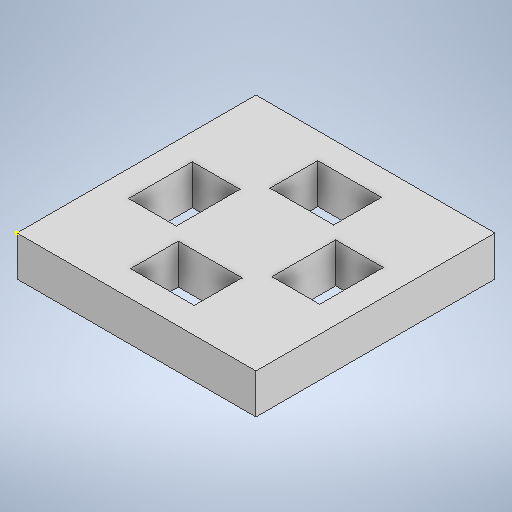
# Autodesk Inventor part: switch_test_v1
Saved by Autodesk Inventor 2025.4 (Build 294407000, 407)
## iProperties
Created: 2026-07-26
Part Number: switch_test_v1
Material: Generic
Document SubType Name: Modeling
Designer: Franchesca
Density: 1 g/cm^3
Appearance: Default
Author: Franchesca
Autodesk Inventor part; units mm, degrees
ref_plane "YZ Plane" through (0, 0, 0) normal (1, 0, 0) x (0, 1, 0)
ref_plane "XZ Plane" through (0, 0, 0) normal (0, 1, 0) x (-1, 0, 0)
ref_plane "XY Plane" through (0, 0, 0) normal (0, 0, 1) x (1, 0, 0)
sketch "Sketch1" plane through (0, 0, 0) normal (0, 1, 0) x (-1, 0, 0)
  point P0 (0, 0)
sketch "Sketch2" plane through (0, 0, 0) normal (0, 1, 0) x (-1, 0, 0)
  line L0 (0, 0) -> (-30, 0)
  line L1 (-30, 0) -> (-30, -30)
  line L2 (-30, -30) -> (0, -30)
  line L3 (0, -30) -> (0, 0)
  line L4 (0, -30) -> (-30, 0) construction
  line L5 (0, 0) -> (-30, -30) construction
  line L6 (-15, -15) -> (0, -15) construction
  line L7 (-15, -15) -> (-30, -15) construction
  line L8 (-15, -15) -> (-15, -30) construction
  line L9 (-15, -15) -> (-15, 0) construction
  line L10 (-15, -15) -> (-9.25, -15) construction
  line L11 (-15, -17.4158) -> (-15, -15) construction
  line L12 (-15, -15) -> (-15, -20.75) construction
  line L13 (-15, -15) -> (-15, -9.25) construction
  line L14 (-15, -15) -> (-9.25, -15) construction
  line L15 (-15, -15) -> (-20.75, -15) construction
  line L16 (-15, -20.75) -> (-9.25, -15) construction
  line L17 (-9.25, -15) -> (-9.25, -20.75) construction
  line L18 (-9.25, -20.75) -> (-15, -20.75) construction
  line L19 (-15, -20.75) -> (-20.75, -20.75) construction
  line L20 (-20.75, -20.75) -> (-20.75, -15) construction
  line L21 (-9.25, -15) -> (-9.25, -9.25) construction
  line L22 (-15, -9.25) -> (-9.25, -9.25) construction
  line L23 (-15, -9.25) -> (-20.75, -9.25) construction
  line L24 (-20.75, -9.25) -> (-20.75, -15) construction
  line L25 (-15, -9.25) -> (-11, -9.25) construction
  line L26 (-15, -9.25) -> (-19, -9.25) construction
  line L27 (-11, -9.25) -> (-19, -9.25)
  line L28 (-11, -9.25) -> (-11, -3.25)
  line L29 (-11, -3.25) -> (-19, -3.25)
  line L30 (-19, -3.25) -> (-19, -9.25)
  line L31 (-11, -20.75) -> (-19, -20.75)
  line L32 (-19, -20.75) -> (-19, -26.75)
  line L33 (-19, -26.75) -> (-11, -26.75)
  line L34 (-11, -26.75) -> (-11, -20.75)
  line L35 (-9.25, -9.25) -> (-9.25, -10.75)
  line L36 (-9.25, -20.75) -> (-9.25, -18.75)
  line L37 (-9.25, -18.75) -> (-9.25, -19.25)
  line L38 (-9.25, -18.75) -> (-9.25, -10.75)
  line L39 (-9.25, -10.75) -> (-3.25, -10.75)
  line L40 (-3.25, -10.75) -> (-3.25, -18.75)
  line L41 (-3.25, -18.75) -> (-9.25, -18.75)
  line L42 (-9.25, -19.25) -> (-20.75, -19.25) construction
  line L43 (-20.75, -19.25) -> (-20.75, -11.25)
  line L44 (-20.75, -11.25) -> (-26.75, -11.25)
  line L45 (-26.75, -11.25) -> (-26.75, -19.25)
  line L46 (-26.75, -19.25) -> (-20.75, -19.25)
  line L47 (-9.25, -18.75) -> (-11.75, -18.75) construction
  line L48 (-11.75, -18.75) -> (-11.75, -10.75) construction
  line L49 (-11.75, -10.75) -> (-9.25, -10.75) construction
  line L50 (-20.75, -19.25) -> (-18.25, -19.25) construction
  line L51 (-18.25, -19.25) -> (-18.25, -11.25) construction
  line L52 (-18.25, -11.25) -> (-20.75, -11.25) construction
  line L53 (-9.25, -10.75) -> (-9.25, -11.75) construction
  line L54 (-9.25, -11.75) -> (-11.75, -11.75) construction
  line L55 (-20.75, -11.25) -> (-20.75, -11.75) construction
  line L56 (-20.75, -11.75) -> (-18.25, -11.75) construction
  line L57 (-11.75, -18.75) -> (-20.75, -18.75) construction
  line L58 (-18.25, -18.75) -> (-18.25, -11.75) construction
  line L59 (-15, -18.75) -> (-14.25, -18.75) construction
  line L60 (-15, -18.75) -> (-15.75, -18.75) construction
  line L61 (-11.75, -18.75) -> (-11.75, -11.75)
  line L62 (-11.75, -18.75) -> (-14.25, -18.75)
  line L63 (-11.75, -11.75) -> (-14.25, -11.75)
  line L64 (-14.25, -18.75) -> (-14.25, -11.75)
  line L65 (-15.75, -18.75) -> (-18.25, -18.75)
  line L66 (-18.25, -18.75) -> (-18.25, -11.75)
  line L67 (-18.25, -11.75) -> (-15.75, -11.75)
  line L68 (-15.75, -11.75) -> (-15.75, -18.75)
  dimension "d0" = 30
  dimension "d1" = 30
  dimension "d3" = 5.75
  dimension "d4" = 5.75
  dimension "d5" = 5.75
  dimension "d6" = 5.75
  dimension "d7" = 4
  dimension "d8" = 4
  dimension "d9" = 6
  dimension "d10" = 6
  dimension "d11" = 8
  dimension "d12" = 1.5
  dimension "d13" = 2
  dimension "d14" = 0.5
  dimension "d15" = 6
  dimension "d16" = 8
  dimension "d17" = 6
  dimension "d18" = 2.5
  dimension "d19" = 2.5
  dimension "d20" = 1
  dimension "d21" = 0.75
  dimension "d22" = 0.75
  constraints: 138 end point, 40 point on line, 17 perpendicular, 5 collinear, 5 midpoint, 4 horizontal, 4 vertical, 3 parallel
  measures "d0" distance of L2.end L1.end
  measures "d1" distance between parallel lines of L0 L2
  measures "d3" distance of L6.start L12.end
  measures "d4" distance of L6.start L13.end
  measures "d5" distance of L6.start L10.end
  measures "d6" distance of L6.start L15.end
  measures "d7" distance of L13.end L25.end
  measures "d8" distance of L13.end L26.end
  measures "d9" distance of L25.end L28.end
  measures "d10" distance of L31.end L32.end
  measures "d11" distance of L25.end L26.end
  measures "d12" distance of L21.end L35.end
  measures "d13" distance of L17.end L36.end
  measures "d14" distance of L36.end L37.end
  measures "d15" distance of L35.end L39.end
  measures "d16" distance of L42.end L43.end
  measures "d17" distance of L43.end L44.end
  measures "d18" distance of L36.end L47.end
  measures "d19" distance of L42.end L50.end
  measures "d20" distance of L35.end L53.end
  measures "d21" distance of L59.start L59.end
  measures "d22" distance of L59.start L60.end
extrude "Extrusion1" add sketch "Sketch2" against normal blind 5
extrude "Extrusion2" add sketch "Sketch2" against normal blind 2.5 contours L62 L64 L63 L61 | L65 L66 L67 L68
body "Solid1"
